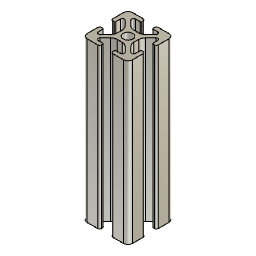
aluminium extrusie 20x20x70mm v1 (Autodesk Fusion 360 archive; units mm, degrees)
design "aluminium extrusie 20x20x70mm" references "aluminium extrusie 20x20x2mm"
Autodesk Fusion 360 part; units mm, degrees
derive "Sketch1" from "Aluminium Extrusie 20x20x2mm v3"
sketch "sketch 190" plane through (0, 0, 0) normal (0, 0, 1) x (-1, 0, 0)
  arc A0 (-4.9118, 8.2) -> (-5.5045, 6.7691) centre (-4.9118, 7.3618) ccw
  line L0 (-4.9118, 8.2) -> (-2.8048, 8.2)
  arc A1 (-2.8048, 8.2) -> (-2.5, 8.5048) centre (-2.8048, 8.5048) ccw
  line L1 (-2.5, 8.5048) -> (-2.5, 9.2126)
  arc A2 (-2.5, 9.2126) -> (-3.2874, 10) centre (-3.2874, 9.2126) ccw
  line L2 (-3.2874, 10) -> (-8, 10)
  arc A3 (-8, 10) -> (-10, 8) centre (-8, 8) ccw
  line L3 (-10, 8) -> (-10, 3.2874)
  arc A4 (-10, 3.2874) -> (-9.2126, 2.5) centre (-9.2126, 3.2874) ccw
  line L4 (-9.2126, 2.5) -> (-8.5048, 2.5)
  arc A5 (-8.5048, 2.5) -> (-8.2, 2.8048) centre (-8.5048, 2.8048) ccw
  line L5 (-8.2, 2.8048) -> (-8.2, 4.9118)
  arc A6 (-6.7691, 5.5045) -> (-8.2, 4.9118) centre (-7.3618, 4.9118) ccw
  line L6 (-6.7691, 5.5045) -> (-4.4787, 3.2141)
  arc A7 (-3.6, 1.0928) -> (-4.4787, 3.2141) centre (-6.6, 1.0928) ccw
  line L7 (-3.6, 1.0928) -> (-3.6, -1.0928)
  arc A8 (-4.4787, -3.2141) -> (-3.6, -1.0928) centre (-6.6, -1.0928) ccw
  line L8 (-4.4787, -3.2141) -> (-6.7691, -5.5045)
  arc A9 (-8.2, -4.9118) -> (-6.7691, -5.5045) centre (-7.3618, -4.9118) ccw
  line L9 (-8.2, -4.9118) -> (-8.2, -2.8048)
  arc A10 (-8.2, -2.8048) -> (-8.5048, -2.5) centre (-8.5048, -2.8048) ccw
  line L10 (-8.5048, -2.5) -> (-9.2126, -2.5)
  arc A11 (-9.2126, -2.5) -> (-10, -3.2874) centre (-9.2126, -3.2874) ccw
  line L11 (-10, -3.2874) -> (-10, -8)
  arc A12 (-10, -8) -> (-8, -10) centre (-8, -8) ccw
  line L12 (-8, -10) -> (-3.2874, -10)
  arc A13 (-3.2874, -10) -> (-2.5, -9.2126) centre (-3.2874, -9.2126) ccw
  line L13 (-2.5, -9.2126) -> (-2.5, -8.5048)
  arc A14 (-2.5, -8.5048) -> (-2.8048, -8.2) centre (-2.8048, -8.5048) ccw
  line L14 (-2.8048, -8.2) -> (-4.9118, -8.2)
  arc A15 (-5.5045, -6.7691) -> (-4.9118, -8.2) centre (-4.9118, -7.3618) ccw
  line L15 (-5.5045, -6.7691) -> (-3.2141, -4.4787)
  arc A16 (-1.0928, -3.6) -> (-3.2141, -4.4787) centre (-1.0928, -6.6) ccw
  line L16 (-1.0928, -3.6) -> (1.0928, -3.6)
  arc A17 (3.2141, -4.4787) -> (1.0928, -3.6) centre (1.0928, -6.6) ccw
  line L17 (3.2141, -4.4787) -> (5.5045, -6.7691)
  arc A18 (4.9118, -8.2) -> (5.5045, -6.7691) centre (4.9118, -7.3618) ccw
  line L18 (4.9118, -8.2) -> (2.8048, -8.2)
  arc A19 (2.8048, -8.2) -> (2.5, -8.5048) centre (2.8048, -8.5048) ccw
  line L19 (2.5, -8.5048) -> (2.5, -9.2126)
  arc A20 (2.5, -9.2126) -> (3.2874, -10) centre (3.2874, -9.2126) ccw
  line L20 (3.2874, -10) -> (8, -10)
  arc A21 (8, -10) -> (10, -8) centre (8, -8) ccw
  line L21 (10, -8) -> (10, -3.2874)
  arc A22 (10, -3.2874) -> (9.2126, -2.5) centre (9.2126, -3.2874) ccw
  line L22 (9.2126, -2.5) -> (8.5048, -2.5)
  arc A23 (8.5048, -2.5) -> (8.2, -2.8048) centre (8.5048, -2.8048) ccw
  line L23 (8.2, -2.8048) -> (8.2, -4.9118)
  arc A24 (6.7691, -5.5045) -> (8.2, -4.9118) centre (7.3618, -4.9118) ccw
  line L24 (6.7691, -5.5045) -> (4.4787, -3.2141)
  arc A25 (3.6, -1.0928) -> (4.4787, -3.2141) centre (6.6, -1.0928) ccw
  line L25 (3.6, -1.0928) -> (3.6, 1.0928)
  arc A26 (4.4787, 3.2141) -> (3.6, 1.0928) centre (6.6, 1.0928) ccw
  line L26 (4.4787, 3.2141) -> (6.7691, 5.5045)
  arc A27 (8.2, 4.9118) -> (6.7691, 5.5045) centre (7.3618, 4.9118) ccw
  line L27 (8.2, 4.9118) -> (8.2, 2.8048)
  arc A28 (8.2, 2.8048) -> (8.5048, 2.5) centre (8.5048, 2.8048) ccw
  line L28 (8.5048, 2.5) -> (9.2126, 2.5)
  arc A29 (9.2126, 2.5) -> (10, 3.2874) centre (9.2126, 3.2874) ccw
  line L29 (10, 3.2874) -> (10, 8)
  arc A30 (10, 8) -> (8, 10) centre (8, 8) ccw
  line L30 (8, 10) -> (3.2874, 10)
  arc A31 (3.2874, 10) -> (2.5, 9.2126) centre (3.2874, 9.2126) ccw
  line L31 (2.5, 9.2126) -> (2.5, 8.5048)
  arc A32 (2.5, 8.5048) -> (2.8048, 8.2) centre (2.8048, 8.5048) ccw
  line L32 (2.8048, 8.2) -> (4.9118, 8.2)
  arc A33 (5.5045, 6.7691) -> (4.9118, 8.2) centre (4.9118, 7.3618) ccw
  line L33 (5.5045, 6.7691) -> (3.2141, 4.4787)
  arc A34 (1.0928, 3.6) -> (3.2141, 4.4787) centre (1.0928, 6.6) ccw
  line L34 (1.0928, 3.6) -> (-1.0928, 3.6)
  arc A35 (-3.2141, 4.4787) -> (-1.0928, 3.6) centre (-1.0928, 6.6) ccw
  line L35 (-3.2141, 4.4787) -> (-5.5045, 6.7691)
  circle A36 centre (0, 0) radius 2.15
extrude "Extrude1" add sketch "sketch 190" along normal mid plane 70
